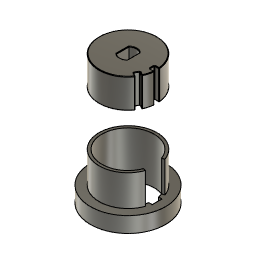
Zemismart 30mm Tube (Autodesk Fusion 360 design; units mm, degrees)
Autodesk Fusion 360 part; units mm, degrees
note: some values were not read from the file. Set by a fixed rule: which sketch regions a step uses.
sketch "Sketch1" plane through (0, 0, 0) normal (0, 0, 1) x (1, 0, 0) in component "Motor Attach"
  circle A0 centre (0, 0) radius 14.9
  circle A1 centre (0, 0) radius 12.375 construction
  circle A2 centre (0, 0) radius 4.25
  line L0 (0, 0) -> (2.75, 0) construction
  line L1 (0, 0) -> (-2.75, 0) construction
  line L2 (-2.75, 0) -> (-2.75, 3.2404)
  line L3 (-2.75, 0) -> (-2.75, -3.2404)
  line L4 (2.75, 0) -> (2.75, -3.2404)
  line L5 (2.75, 0) -> (2.75, 3.2404)
  circle A3 centre (0, 0) radius 9.125
  dimension "d1" = 29.8
  dimension "d4" = 24.75
  dimension "d7" = 8.5
  dimension "d8" = 2.75
  dimension "d9" = 2.75
  dimension "d12" = 18.25
  constraint coincident A0.centre A1.centre
  constraint concentric A1 A2
  constraint horizontal L0
  constraint parallel L0 L1
  constraint coincident A2 L2.end
  constraint perpendicular L1 L2
  constraint coincident A2 L3.end
  constraint perpendicular L1 L3
  constraint coincident A2 L4.end
  constraint perpendicular L0 L4
  constraint coincident A2 L5.end
  constraint perpendicular L0 L5
  constraint concentric A2 A3
  measures "d1" diameter of A0
  measures "d4" diameter of A1
  measures "d7" diameter of A2
  measures "d8" distance of A0.centre L0.end
  measures "d9" distance of A0.centre L1.end
  measures "d12" diameter of A3
extrude "Extrude1" add sketch "Sketch1" along normal blind 15.25 contours A0 | A2 L4 L5 | A2 L2 L3 | A3 makes body 1 in component "Motor Attach"
extrude "Extrude2" cut sketch "Sketch1" against normal blind 5 from surface at 15.25 contours A2 L4 L5 | A2 L2 L3 | A3 bodies 1 in component "Motor Attach"
fillet "Fillet1" radius 0.25 3 faces at (-4.875, 0, 10.25) (9.1137, -0.4548, 11.9167) (12.9195, -0.7402, 15.25) on bodies 1 in component "Motor Attach"
fillet "Fillet2" radius 0.25 1 faces at (-6.8, 0, 0) on bodies 1 in component "Motor Attach"
sketch "Sketch1 (2)" plane through (0, 0, 0) normal (0, 0, 1) x (1, 0, 0) in component "Motor Ring"
  circle A0 centre (0, 0) radius 17.875
  line L0 (-9.0114, 15.4373) -> (8.9886, 15.4506)
  line L1 (-9.0114, 15.4373) -> (-5.0783, 15.4373) construction
  circle A1 centre (0, 0) radius 2.5 construction
  line L2 (-17.6993, 2.5) -> (17.6993, 2.5) construction
  line L3 (-9.0114, 15.4373) -> (-1.5421, 2.5)
  line L4 (-9.0114, 15.4373) -> (-5.4753, 15.4373) construction
  line L5 (8.9886, 15.4506) -> (1.5115, 2.5)
  line L6 (8.9886, 15.4506) -> (12.5579, 15.4506) construction
  line L7 (1.5115, 2.5) -> (-1.5421, 2.5)
  dimension "d1_1" = 35.75
  dimension "d2_1" = 18
  dimension "d4_1" = 5
  dimension "d5_1" = 60
  dimension "d6_1" = 120
  constraint coincident A0.centre A1.centre
  constraint coincident A0 L0.start
  constraint coincident A0 L0.end
  constraint horizontal L1
  constraint coincident A0 L2.start
  constraint coincident A0 L2.end
  constraint horizontal L2
  constraint tangent A1 L2
  constraint horizontal L4
  constraint coincident L2 L3.end
  constraint horizontal L6
  constraint coincident L2 L5.end
  measures "d1_1" diameter of A0
  measures "d2_1" distance of L0.start L0.end
  measures "d4_1" diameter of A1
  measures "d5_1" angle of L3 L4
  measures "d6_1" angle of L5 L6
sketch "Ring Base" plane through (0, 0, 0) normal (0, 0, 1) x (1, 0, 0) in component "Motor Ring"
  circle A0 centre (0, 0) radius 19.375
  circle A1 centre (0, 0) radius 13.5
  line L0 (15, 2.5) -> (-15, 2.5)
  line L1 (-15, 2.5) -> (-15, -2.5)
  line L2 (-15, -2.5) -> (15, -2.5)
  line L3 (15, -2.5) -> (15, 2.5)
  line L4 (15, 2.5) -> (-15, -2.5) construction
  line L5 (-15, 2.5) -> (15, -2.5) construction
  dimension "d18" = 38.75
  dimension "d19" = 27
  dimension "d20" = 30
  dimension "d21" = 5
  constraint coincident A0.centre A1.centre
  constraint horizontal L0
  constraint perpendicular L0 L1
  constraint parallel L0 L2
  constraint parallel L1 L3
  constraint coincident L4 A0.centre
  constraint coincident L5 A0.centre
  measures "d18" diameter of A0
  measures "d19" diameter of A1
  measures "d20" distance of L1.end L2.end
  measures "d21" distance of L0.end L1.end
extrude "Extrude1'" add sketch "Ring Base" along normal blind 8 separate body contours A0 | A1 L0 L1 L2 makes body 2 in component "Motor Ring"
sketch "Sketch2" plane through (0, 0, 0) normal (0, 0, 1) x (1, 0, 0)
sketch "Sketch2 (2)" plane through (0, 0, 0) normal (0, 0, 1) x (1, 0, 0) in component "Motor Attach"
  circle A0 centre (0, 0) radius 14.9
  line L0 (0, 0) -> (14.9, 0)
  line L1 (0, 0) -> (14.9, 0) construction
  line L2 (0, 0) -> (14.9, 0) construction
  line L3 (0, 0) -> (12.9038, 7.45)
  line L4 (0, 0) -> (14.9, 0) construction
  line L5 (0, 0) -> (14.3923, 3.8564) construction
  line L6 (0, 0) -> (14.9, 0) construction
  line L7 (14.9, 0) -> (12.4, 0)
  line L8 (12.4, 0) -> (12.4, -1)
  line L9 (12.65, -1.25) -> (14.8475, -1.25)
  arc A1 (12.4, -1) -> (12.65, -1.25) centre (12.65, -1) ccw
  line L10 (12.4, 0) -> (12.4, 1)
  arc A2 (12.65, 1.25) -> (12.4, 1) centre (12.65, 1) ccw
  line L11 (12.65, 1.25) -> (14.8475, 1.25)
  line L12 (11.5802, 5.2425) -> (13.4833, 6.3412)
  arc A3 (11.2387, 5.334) -> (11.5802, 5.2425) centre (11.4552, 5.459) ccw
  line L13 (10.7387, 6.2) -> (11.2387, 5.334)
  line L14 (10.7387, 6.2) -> (10.2387, 7.066)
  arc A4 (10.3302, 7.4075) -> (10.2387, 7.066) centre (10.4552, 7.191) ccw
  line L15 (10.3302, 7.4075) -> (12.2333, 8.5063)
  point P0 (12.4, -1.25)
  dimension "d57" = 14.9
  dimension "d58" = 30
  dimension "d59" = 14.9
  dimension "d60" = 15
  dimension "d65" = 2.5
  dimension "d66" = 1.25
  dimension "d67" = 0.25
  constraint coincident A0.centre L0.start
  constraint coincident A0 L0.end
  constraint horizontal L0
  constraint horizontal L1
  constraint horizontal L2
  constraint horizontal L4
  constraint horizontal L6
  constraint parallel L4 L7
  constraint perpendicular L4 L8
  constraint horizontal L9
  constraint coincident P0 L8
  constraint coincident P0 L9
  constraint tangent L8 A1
  constraint tangent L9 A1
  constraint symmetric L1 L7.end L8.start
  constraint symmetric L1 L9.end L11.end
  constraint symmetric L1 L8.end L10.end
  constraint symmetric L1 L9.start A2.start
  constraint symmetric L1 A1 A2
  constraint symmetric L5 L7.end L13.start
  constraint symmetric L5 L9.end L15.end
  constraint symmetric L5 L8.end L14.end
  constraint symmetric L5 L9.start A4.start
  constraint symmetric L5 A1 A4
  constraint symmetric L5 L10.end A3.start
  constraint symmetric L5 A2.start L12.start
  constraint symmetric L5 A2 A3
  constraint symmetric L5 L11.end L12.end
  measures "d57" distance of A0.centre L3.end
  measures "d58" angle of L3 L4
  measures "d59" distance of A0.centre L5.end
  measures "d60" angle of L5 L6
  measures "d65" distance of L0.end L7.end
  measures "d66" distance of L7.end P0
  measures "d67" radius of A1
extrude "Extrude4" cut sketch "Sketch2 (2)" along normal blind 20 contours A0 L0 L7 L10 A2 L11 | A0 L0 L7 L8 L9 A1 | A0 L3 L12 A3 L13 | A0 L3 L14 A4 L15 bodies 1 in component "Motor Attach"
fillet "Fillet3" radius 0.25 32 edges at (13.6233, 1.25, 15.25) (14.7738, 1.25, 15.1769) (14.8475, 1.25, 7.625) (14.7738, 1.25, 0.0731) (13.6233, 1.25, 0) (12.4732, 1.1768, 0) (12.4, 0, 0) (12.4732, -1.1768, 0) (13.6233, -1.25, 0) (14.7738, -1.25, 0.0731) (14.8475, -1.25, 7.625) (14.7738, -1.25, 15.1769) (13.6233, -1.25, 15.25) (12.4732, -1.1768, 15.25) (12.4, 0, 15.25) (12.4732, 1.1768, 15.25) (11.1731, 7.8942, 15.25) (12.1695, 8.4695, 15.1769) (12.2333, 8.5063, 7.625) (12.1695, 8.4695, 0.0731) (11.1731, 7.8942, 0) (10.2137, 7.2557, 0) (10.7387, 6.2, 0) (11.3905, 5.2175, 0) (12.4231, 5.7291, 0) (13.4195, 6.3044, 0.0731) (13.4833, 6.3412, 7.625) (13.4195, 6.3044, 15.1769) (12.4231, 5.7291, 15.25) (11.3905, 5.2175, 15.25) (10.7387, 6.2, 15.25) (10.2137, 7.2557, 15.25) on bodies 1 in component "Motor Attach"
extrude "Extrude4'" add sketch "Sketch2 (2)" along normal blind 16 from surface at 8 separate body contours A0 L0 L3 L10 A2 L11 L12 A3 L13 | A0 L0 L3 L8 L9 A1 L14 A4 L15 makes body 3 in component "Motor Ring"
move_body "Move4" bodies 3 to x (0.965926, -0.258819, 0) y (0.258819, 0.965926, 0) z (0, 0, 1) at (0, 0, 0) in component "Motor Ring"
extrude "Extrude5" cut sketch "Ring Base" along normal blind 24 contours A1 L0 L2 | A1 L0 L2 L3 | A1 L0 | A1 L2 bodies 3 makes body 4 at (14.5124, 2.5, 18.6667) makes body 5 at (13.456, -6.3989, 13.3333) in component "Motor Ring"
combine "Combine1" operation add target body 2 tool bodies 5 in component "Motor Ring"
move_body "Move1" bodies 1 to x (1, 0, 0) y (0, -1, 0) z (0, 0, -1) at (0, 0, 0) in component "Motor Attach"
move_body "Move2" bodies 1 to x (1, 0, 0) y (0, 1, 0) z (0, 0, 1) at (0, 0, 67) in component "Motor Attach"
move_body "Move3" [rolled back] rotate angle -90 in component "Motor Attach"
move_body "Move4'" [rolled back] in component "Motor Attach"
component "Motor Attach" placed x (1, 0, 0) y (0, 1, 0) z (0, 0, 1) at (0, 0, 0)
component "Motor Ring" placed x (1, 0, 0) y (0, 1, 0) z (0, 0, 1) at (0, 0, 0)
hidden bodies 3 4
equation "d57 = ( 29.8 / 2 ) * 1 mm"
equation "d59 = ( 29.8 / 2 ) * 1 mm"
named bodies: "Motor Attachment", "Motor Ring"
